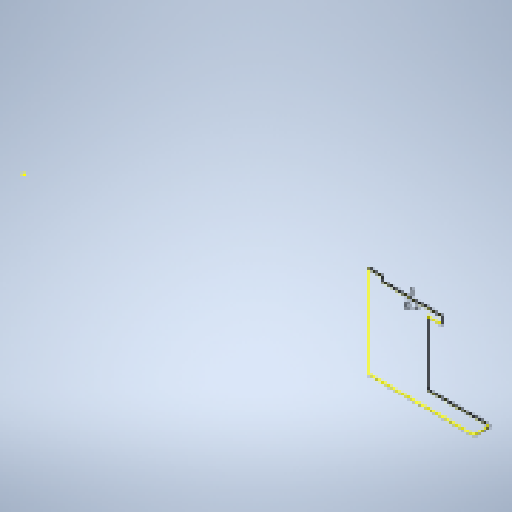
# Autodesk Inventor part: X-Motor Jig v0.1
Saved by Autodesk Inventor 2023 (Build 270158000, 158)
## iProperties
Created: 2023-07-27
Part Number: X-Motor Jig v0.1
Material: Generic
Document SubType Name: Modeling
Designer: Parker
Density: 1 g/cm^3
Appearance: Default
Author: Parker
Autodesk Inventor part; units mm, degrees
ref_plane "YZ Plane" through (0, 0, 0) normal (1, 0, 0) x (0, 1, 0)
ref_plane "XZ Plane" through (0, 0, 0) normal (0, 1, 0) x (-1, 0, 0)
ref_plane "XY Plane" through (0, 0, 0) normal (0, 0, 1) x (1, 0, 0)
sketch "Sketch1" plane through (0, 0, 0) normal (0, 0, 1) x (1, 0, 0)
  line L0 (281, 55.5) -> (291, 55.5) projected
  line L1 (281, 55.5) -> (281, 11) projected
  line L2 (281, 11) -> (323.5, 11) projected
  line L3 (323.5, 11) -> (323.5, 10) projected
  line L4 (313.5, 0) -> (323.5, 10) projected
  line L5 (313.5, 0) -> (240, 0) projected
  line L6 (240, 63.75) -> (240, 0) projected
  line L7 (250, 63.75) -> (240, 63.75) projected
  line L8 (250, 60.5) -> (250, 63.75) projected
  line L9 (291, 60.5) -> (250, 60.5) projected
  line L10 (291, 60.5) -> (291, 55.5) projected
  line L11 (250.2, 60.7) -> (250.2, 63.95)
  line L12 (250.2, 63.95) -> (239.8, 63.95)
  line L13 (239.8, 63.95) -> (239.8, -0.2)
  line L14 (239.8, -0.2) -> (313.5828, -0.2)
  line L15 (313.5828, -0.2) -> (323.7, 9.9172)
  line L16 (323.7, 9.9172) -> (323.7, 11.2)
  line L17 (323.7, 11.2) -> (281.2, 11.2)
  line L18 (281.2, 11.2) -> (281.2, 55.3)
  line L19 (281.2, 55.3) -> (291.2, 55.3)
  line L20 (291.2, 55.3) -> (291.2, 60.7)
  line L21 (291.2, 60.7) -> (250.2, 60.7)
  line L22 (333.7, -10.2) -> (239.8, -10.2)
  line L23 (239.8, -10.2) -> (239.8, 70.7)
  line L24 (239.8, 70.7) -> (333.7, 70.7)
  line L25 (333.7, 70.7) -> (333.7, -10.2)
  line L26 (239.8, 70.7) -> (214.8, 70.7)
  line L27 (214.8, 70.7) -> (214.8, -10.2)
  line L28 (214.8, -10.2) -> (239.8, -10.2)
  line L29 (239.8, -10.2) -> (239.8, 70.7)
  line L30 (291, 22.5) -> (291, 54) projected
  line L31 (296.8211, 22.5) -> (291, 22.5) projected
  arc A0 (296.8211, 22.5) -> (308.1789, 22.5) centre (302.5, 32.5) ccw projected
  line L32 (323.5, 22.5) -> (308.1789, 22.5) projected
  line L33 (323.5, 11) -> (323.5, 22.5) projected
  line L34 (281, 11) -> (323.5, 11) projected
  line L35 (281, 54) -> (281, 11) projected
  line L36 (291, 54) -> (281, 54) projected
  circle A1 centre (287, 17) radius 1.6 projected
  circle A2 centre (318, 17) radius 1.6 projected
  circle A3 centre (287, 48) radius 1.6 projected
  line L37 (280.8, 11) -> (280.8, 54.2)
  line L38 (280.8, 54.2) -> (291.2, 54.2)
  line L39 (291.2, 54.2) -> (291.2, 22.7)
  line L40 (291.2, 22.7) -> (296.8742, 22.7)
  arc A4 (296.8742, 22.7) -> (308.1258, 22.7) centre (302.5, 32.5) ccw
  line L41 (308.1258, 22.7) -> (323.7, 22.7)
  line L42 (323.7, 22.7) -> (323.7, 11)
  line L43 (291.2, 54.2) -> (291.2, 55.3)
  point P0 (0, 0)
  point P1 (276.6914, -0.2)
  point P2 (323.7, 10.5586)
  point P3 (323.7, 11.0919)
  dimension "d0" = 0.2
  dimension "d1" = 10
  dimension "d2" = 0
  dimension "d3" = 10
  dimension "d4" = 10
  dimension "d5" = 25
  dimension "d6" = 0.2
  constraints: 52 end point, 4 parallel, 2 horizontal, 2 midpoint, 2 perpendicular, 2 point on circle, 1 centre point, 16 other
  measures "d0" distance between parallel lines of L9 L21
  measures "d1" distance from line of point (276.691, -0.2) L22
  measures "d2" distance between parallel lines of L23 L13
  measures "d3" distance between parallel lines of L21 L24
  measures "d4" distance from line of point (323.7, 10.559) L25
  measures "d5" distance of L22.end L27.end
  measures "d6" distance between parallel lines of L32 L41
extrude "Extrusion1" add sketch "Sketch1" along normal blind 15 contours L43 L20 L21 L11 L12 L23 L24 L25 L22 L14 L15 L16 L42 L41 A4 L40 L39
sketch "Sketch2" plane through (0, 0, 0) normal (0, 0, 1) x (1, 0, 0)
  line L0 (239.8, 70.7) -> (239.8, -10.2) projected
  line L1 (214.8, -10.2) -> (239.8, -10.2) projected
  line L2 (214.8, 70.7) -> (214.8, -10.2) projected
  line L3 (239.8, 70.7) -> (214.8, 70.7) projected
  point P0 (0, 0)
ref_plane "Work Plane1" through (-211.5, 59.3125, 19.5) normal (0, 0, 1) x (1, 0, 0)
extrude "Extrusion2" add sketch "Sketch2" along normal up to surface (19.5 mm away)
sketch "Sketch3" plane through (0, 0, 0) normal (0, 0, -1) x (-1, 0, 0)
  line L0 (-214.8, -10.2) -> (-333.7, -10.2) projected
  line L1 (-333.7, 70.7) -> (-214.8, 70.7) projected
  line L2 (-333.7, -10.2) -> (-214.8, -10.2)
  line L3 (-214.8, -10.2) -> (-214.8, 70.7)
  line L4 (-214.8, 70.7) -> (-333.7, 70.7)
  line L5 (-333.7, 70.7) -> (-333.7, -10.2)
  point P0 (0, 0)
  point P1 (-214.8, -10.2)
  constraints: 8 end point, 2 parallel, 1 horizontal, 1 perpendicular
ref_plane "Work Plane2" through (240, 0, 7.5) normal (0, 0, -1) x (0, 1, 0)
extrude "Extrusion3" add sketch "Sketch3" against normal up to surface (7.5 mm away)
sketch "Sketch4" plane through (0, 0, 0) normal (0, 0, -1) x (-1, 0, 0)
  line L0 (-333.7, -10.2) -> (-333.7, 70.7) projected
  line L1 (-333.7, 70.7) -> (-214.8, 70.7)
  line L2 (-214.8, 70.7) -> (-214.8, 90.7)
  line L3 (-214.8, 90.7) -> (-333.7, 90.7)
  line L4 (-333.7, 90.7) -> (-333.7, 70.7)
  line L5 (-333.7, -10.2) -> (-214.8, -10.2)
  line L6 (-214.8, -10.2) -> (-214.8, -30.2)
  line L7 (-214.8, -30.2) -> (-333.7, -30.2)
  line L8 (-333.7, -30.2) -> (-333.7, -10.2)
  point P0 (0, 0)
  dimension "d13" = 20
  dimension "d14" = 20
  constraints: 16 end point, 4 parallel, 2 horizontal, 2 perpendicular, 1 point on line
  measures "d13" distance of L7.end L0.start
  measures "d14" distance of L3.end L0.end
ref_plane "Work Plane3" through (-297.2, 78.7, 10) normal (0, 0, 1) x (1, 0, 0)
extrude "Extrusion4" add sketch "Sketch4" against normal up to surface (10 mm away)
sketch "Sketch5" plane through (214.8, -10.2, 19.5) normal (-1, 0, 0) x (0, 0, 1)
  circle A0 centre (0, 62.7) radius 5 projected
  circle A1 centre (0, 17.7) radius 5 projected
  circle A2 centre (0, 62.7) radius 5.1
  circle A3 centre (0, 17.7) radius 5.1
  point P0 (-19.5, 10.2)
  dimension "d17" = 0.1
  dimension "d18" = 0.1
  constraints: 2 centre point
  measures "d17" radial gap between concentric circles of A0 A2
  measures "d18" radial gap between concentric circles of A1 A3
extrude "Extrusion5" cut sketch "Sketch5" against normal up to surface (25 mm away) contours A0 | A1 | A2 | A3
sketch "Sketch6" plane through (214.8, 90.7, 10) normal (0, 0, 1) x (1, 0, 0)
  line L0 (10, -10) -> (108.9, -10)
  line L1 (108.9, -10) -> (108.9, -110.9)
  line L2 (108.9, -110.9) -> (10, -110.9)
  line L3 (10, -110.9) -> (10, -10)
  line L4 (118.9, -100.9) -> (118.9, -120.9) projected
  line L5 (118.9, -120.9) -> (0, -120.9) projected
  line L6 (0, 0) -> (118.9, 0) projected
  line L7 (0, -20) -> (0, 0) projected
  point P0 (-214.8, -90.7)
  point P1 (0, -10)
  dimension "d21" = 10
  dimension "d22" = 10
  dimension "d23" = 10
  dimension "d24" = 10
  constraints: 8 end point, 4 coincident, 2 parallel, 1 horizontal, 1 midpoint, 1 perpendicular
  measures "d21" distance from line of L4 L1.end
  measures "d22" distance from line of L5 L1.end
  measures "d23" distance from line of L6 L0.start
  measures "d24" distance of point (0, -10) L0.start
hole "Hole1" at (323.7, -20.2, 10) at (224.8, -20.2, 10) at (224.8, 80.7, 10) at (323.7, 80.7, 10) direction (0, 0, -1) diameter 5.5 end through all counterbore diameter 12.24 counterbore depth 1.5 clearance for "Hex Head Bolt" size "M5" standard "Ansi Metric M Profile"
chamfer "Chamfer1" distance 1 angle 45 11 edges at (276.6914, -0.2, 15) (318.6414, 4.8586, 15) (323.7, 16.8959, 15) (323.7, 10.5045, 15) (315.9129, 22.7, 15) (302.5, 21.2, 15) (294.0371, 22.7, 15) (291.2, 41.7, 15) (270.7, 60.7, 15) (250.2, 62.325, 15) (245, 63.95, 15)
chamfer "Chamfer2" distance 8 angle 45 2 edges at (274.25, -10.2, 10) (274.25, 70.7, 10)
fillet "Fillet1" radius 2 6 edges at (227.3, -10.2, 19.5) (227.3, 2.4, 19.5) (227.3, 12.6, 19.5) (227.3, 47.4, 19.5) (227.3, 57.6, 19.5) (227.3, 70.7, 19.5)
chamfer "Chamfer3" distance 1 angle 45 26 edges at (239.8, 13.1139, 19.1011) (239.8, 30, 19.5) (239.8, 46.8861, 19.1011) (239.8, 52.5, 14.4) (239.8, 58.1139, 19.1011) (239.8, 64.038, 19.5) (239.8, 69.9883, 19.0811) (239.8, 7.5, 14.4) (239.8, 1.8861, 19.1011) (239.8, -3.788, 19.5) (239.8, -9.4883, 19.0811) (214.8, 30, 19.5) (214.8, 46.8861, 19.1011) (214.8, 52.5, 14.4) (214.8, 58.1139, 19.1011) (214.8, 64.038, 19.5) (214.8, 69.9883, 19.0811) (214.8, 13.1139, 19.1011) (214.8, 7.5, 14.4) (214.8, 1.8861, 19.1011) (214.8, -3.788, 19.5) (214.8, -9.4883, 19.0811) (239.8, -11.7, 16.5) (239.8, 72.2, 16.5) (214.8, -14.2, 14) (214.8, 74.7, 14)
fillet "Fillet2" radius 5 4 edges at (214.8, -30.2, 5) (333.7, -30.2, 5) (333.7, 90.7, 5) (214.8, 90.7, 5)
chamfer "Chamfer4" distance 1 angle 45 1 edges at (333.7, 30.25, 15)
chamfer "Chamfer5" distance 1 angle 45 28 edges at (274.25, -30.2, 10) (216.2645, -28.7355, 10) (214.8, -21.7, 10) (214.8, -17.4929, 10) (332.2355, -28.7355, 10) (333.7, -21.7, 10) (274.25, -30.2, 0) (216.2645, -28.7355, 0) (214.8, 30.25, 0) (216.2645, 89.2355, 0) (274.25, 90.7, 0) (332.2355, 89.2355, 0) (333.7, 30.25, 0) (332.2355, -28.7355, 0) (224.8, -17.45, 8.5) (323.7, -17.45, 8.5) (224.8, 83.45, 8.5) (274.25, 90.7, 10) (332.2355, 89.2355, 10) (333.7, 82.2, 10) (216.2645, 89.2355, 10) (214.8, 82.2, 10) (214.8, 77.9929, 10) (323.7, 83.45, 8.5) (224.8, -17.45, 0) (224.8, 83.45, 0) (323.7, 83.45, 0) (323.7, -17.45, 0)
body "Solid1"
